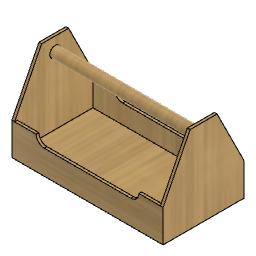
gyakorlati 13 szerszamos lada (Autodesk Fusion 360 design; units mm, degrees)
Autodesk Fusion 360 part; units mm, degrees
sketch "Sketch1" plane through (0, 0, 0) normal (1, 0, 0) x (0, 1, 0)
  line L0 (0, 0) -> (0, 50)
  line L1 (0, 0) -> (125, 0)
  line L2 (125, 0) -> (150, 0)
  line L3 (150, 0) -> (150, 50)
  line L4 (0, 50) -> (50, 150)
  line L5 (50, 150) -> (100, 150)
  line L6 (100, 150) -> (150, 50)
  circle A0 centre (75, 125) radius 10
  constraint coincident L0.start L1.start
  constraint vertical L0
  constraint horizontal L1
  constraint parallel L1 L2
  constraint perpendicular L2 L3
  constraint perpendicular L0 L5
extrude "Extrude1" add sketch "Sketch1" along normal blind 5 makes body 1
ref_plane "WorkPlane1" through (275, 75, 75) normal (1, 0, 0) x (0, 1, 0)
sketch "Sketch2" plane through (275, 75, 75) normal (1, 0, 0) x (0, 1, 0)
  line L0 (-75, -75) -> (-75, -25)
  line L1 (-75, -25) -> (-25, 75)
  line L2 (-25, 75) -> (25, 75)
  line L3 (25, 75) -> (75, -25)
  line L4 (75, -25) -> (75, -75)
  line L5 (75, -75) -> (-75, -75)
  circle A0 centre (0, 50) radius 10
  constraint vertical L0
  constraint perpendicular L0 L2
  constraint perpendicular L2 L4
  constraint perpendicular L0 L5
extrude "Extrude2" add sketch "Sketch2" along normal blind 5 separate body makes body 2
sketch "Sketch3" plane through (0, 0, 0) normal (0, 1, 0) x (1, 0, 0)
  line L0 (5, 0) -> (275, 0)
  line L1 (275, 0) -> (275, -50)
  line L2 (275, -50) -> (235, -50)
  line L3 (235, -50) -> (235, -50)
  line L4 (220, -35) -> (60, -35)
  line L5 (45, -50) -> (45, -50)
  line L6 (45, -50) -> (5, -50)
  line L7 (5, -50) -> (5, 0)
  arc A0 (60, -35) -> (45, -50) centre (60, -50) ccw
  arc A1 (235, -50) -> (220, -35) centre (220, -50) ccw
  dimension "d6" = 15
  dimension "d7" = 15
  constraint horizontal L0
  constraint perpendicular L0 L1
  constraint perpendicular L1 L2
  constraint perpendicular L1 L4
  constraint perpendicular L0 L7
  constraint tangent L4 A0
  constraint tangent L4 A1
  measures "d6" radius of A0
  measures "d7" radius of A1
extrude "Extrude3" add sketch "Sketch3" along normal blind 5 bodies 1 2
ref_plane "WorkPlane2" through (0, 150, 0) normal (0, 1, 0) x (0, 0, 1)
sketch "Sketch4" plane through (0, 150, 0) normal (0, 1, 0) x (1, 0, 0)
  line L0 (5, -50) -> (5, 0)
  line L1 (5, 0) -> (275, 0)
  line L2 (275, 0) -> (275, -50)
  line L3 (275, -50) -> (235, -50)
  line L4 (235, -50) -> (235, -50)
  line L5 (220, -35) -> (60, -35)
  line L6 (45, -50) -> (45, -50)
  line L7 (45, -50) -> (5, -50)
  arc A0 (60, -35) -> (45, -50) centre (60, -50) ccw
  arc A1 (235, -50) -> (220, -35) centre (220, -50) ccw
  dimension "d11" = 15
  dimension "d12" = 15
  constraint vertical L0
  constraint perpendicular L0 L1
  constraint perpendicular L1 L2
  constraint perpendicular L2 L3
  constraint perpendicular L0 L7
  constraint tangent L5 A0
  constraint tangent L5 A1
  measures "d11" radius of A0
  measures "d12" radius of A1
extrude "Extrude4" add sketch "Sketch4" against normal blind 5 bodies 1
sketch "Sketch5" plane through (0, 0, 0) normal (0, 0, 1) x (1, 0, 0)
  line L0 (0, 150) -> (0, 0)
  line L1 (0, 0) -> (280, 0)
  line L2 (280, 0) -> (280, 150)
  line L3 (280, 150) -> (0, 150)
  constraint coincident L0.end L1.start
  constraint vertical L0
  constraint perpendicular L0 L1
  constraint perpendicular L1 L2
  constraint perpendicular L0 L3
extrude "Extrude5" add sketch "Sketch5" against normal blind 10 bodies 1
sketch "Sketch6" plane through (280, 0, 0) normal (1, 0, 0) x (0, 1, 0)
  circle A0 centre (75, 125) radius 10
  line L0 (150, -10) -> (150, 50)
  line L1 (150, 50) -> (100, 150)
  line L2 (100, 150) -> (50, 150)
  line L3 (50, 150) -> (0, 50)
  line L4 (0, 50) -> (0, -10)
  line L5 (0, -10) -> (150, -10)
  circle A1 centre (75, 125) radius 10
  constraint concentric A0 A1
extrude "Extrude6" add sketch "Sketch6" against normal blind 280 contours A0 A1 bodies 1
